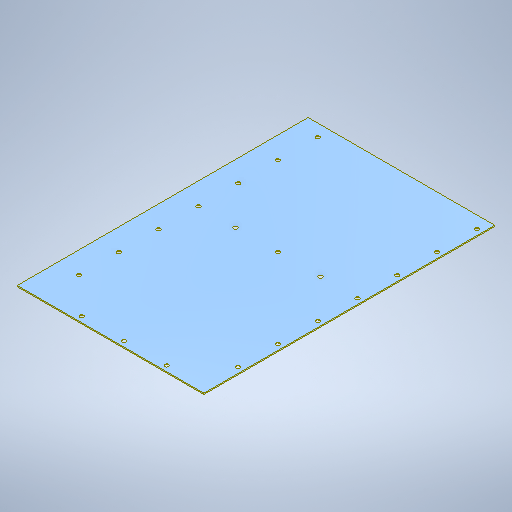
# Autodesk Inventor part: нижняя плита
Saved by Autodesk Inventor 2025 (Build 290162000, 162)
## iProperties
Created: 2025-01-21
Part Number: нижняя плита
Material: СВМПЭ, белый
Document SubType Name: Modeling
Designer: volko
Density: 0.94 g/cm^3
Appearance: Гладкий — белый
Mass: 840.848 g
Surface Area: 3697.01 cm^2
Volume: 894.519 cm^3
Author: volko
Autodesk Inventor part; units mm, degrees
ref_plane "YZ Plane" through (0, 0, 0) normal (1, 0, 0) x (0, 1, 0)
ref_plane "XZ Plane" through (0, 0, 0) normal (0, 1, 0) x (-1, 0, 0)
ref_plane "XY Plane" through (0, 0, 0) normal (0, 0, 1) x (1, 0, 0)
sketch "Эскиз1" plane through (0, 0, 0) normal (0, 1, 0) x (-1, 0, 0)
  line L0 (0, 265) -> (170, 265)
  line L1 (170, 265) -> (170, -265)
  line L2 (0, 265) -> (0, 0)
  line L3 (0, 0) -> (200, 0)
  line L4 (0, 265) -> (-170, 265)
  line L5 (-170, 265) -> (-170, -265)
  line L6 (0, -265) -> (170, -265)
  line L7 (170, -265) -> (170, -125)
  line L8 (-170, -265) -> (-170, -125)
  line L9 (0, -265) -> (-170, -265)
  point P0 (170, 125)
  point P1 (-170, 125)
  dimension "d3" = 340
  dimension "d6" = 530
  constraints: 20 end point, 7 symmetric about line, 4 point on line, 1 vertical
  measures "d3" distance between parallel lines of L5 L1
  measures "d6" distance between parallel lines of L4 L9
extrude "Выдавливание1" add sketch "Эскиз1" along normal blind 2
sketch "Эскиз2" plane through (0, 0, 0) normal (0, 1, 0) x (1, 0, 0)
  line L0 (-170, -265) -> (170, -265) projected
  line L1 (170, -265) -> (170, 265) projected
  point P0 (0, 0)
  point P1 (92.5, -255)
  point P2 (15, -255)
  point P3 (-62.5, -255)
  point P4 (92.5, 25)
  point P5 (15, 25)
  point P6 (-62.5, 25)
  point P7 (92.5, 305)
  point P8 (15, 305)
  point P9 (-62.5, 305)
  point P10 (160, -192.5)
  point P11 (160, -120)
  point P12 (160, -47.5)
  point P13 (160, 25)
  point P14 (160, 97.5)
  point P15 (160, 170)
  point P16 (160, 242.5)
  point P17 (-130, -192.5)
  point P18 (-130, -120)
  point P19 (-130, -47.5)
  point P20 (-130, 25)
  point P21 (-130, 97.5)
  point P22 (-130, 170)
  point P23 (-130, 242.5)
  dimension "d15" = 10
  dimension "d16" = 77.5
  dimension "d19" = 77.5
  dimension "d22" = 280
  dimension "d25" = 10
  dimension "d26" = 72.5
  dimension "d29" = 72.5
  dimension "d32" = 290
  constraints: 2 horizontal, 2 vertical, 21 other
  measures "d15" distance from line of L0 point (92.5, -255)
  measures "d16" distance from line of point (92.5, -255) L1
  measures "d19" distance of point (92.5, -255) point (15, -255)
  measures "d22" distance of point (92.5, -255) point (92.5, 25)
  measures "d25" distance from line of point (160, -192.5) L1
  measures "d26" distance from line of L0 point (160, -192.5)
  measures "d29" distance of point (160, -192.5) point (160, -120)
  measures "d32" distance of point (160, -192.5) point (-130, -192.5)
hole "Отверстие2" at (92.5, 0, 255) at (15, 0, 255) at (-62.5, 0, 255) at (92.5, 0, -25) at (15, 0, -25) at (-62.5, 0, -25) at (92.5, 0, -305) at (15, 0, -305) at (-62.5, 0, -305) at (160, 0, 192.5) at (160, 0, 120) at (160, 0, 47.5) at (160, 0, -25) at (160, 0, -97.5) at (160, 0, -170) at (160, 0, -242.5) at (-130, 0, 192.5) at (-130, 0, 120) at (-130, 0, 47.5) at (-130, 0, -25) at (-130, 0, -97.5) at (-130, 0, -170) at (-130, 0, -242.5) direction (0, 1, 0) diameter 3 end through all countersink diameter 11 countersink angle 90
sketch "Эскиз3" plane through (0, 0, 0) normal (0, -1, 0) x (1, 0, 0)
  line L0 (-238, 0) -> (238, 0) projected
  line L1 (0, -371) -> (0, 371) projected
  line L2 (-170, 265) -> (170, 265) projected
  point P0 (0, 0)
  point P1 (120, 207)
  point P2 (64, 207)
  point P3 (120, 235)
  point P4 (64, 235)
  point P5 (-120, 207)
  point P6 (-64, 207)
  point P7 (-120, 235)
  point P8 (-64, 235)
  point P9 (120, -207)
  point P10 (64, -207)
  point P11 (120, -235)
  point P12 (64, -235)
  point P13 (-120, -235)
  point P14 (-120, -207)
  point P15 (-64, -207)
  point P16 (-64, -235)
  dimension "d52" = 56
  dimension "d55" = 28
  dimension "d59" = 120
  dimension "d60" = 30
  constraints: 12 symmetric about line, 1 horizontal, 1 vertical, 3 other
  measures "d52" distance of point (120, 207) point (64, 207)
  measures "d55" distance of point (120, 207) point (120, 235)
  measures "d59" distance from line of L1 point (120, 207)
  measures "d60" distance from line of L2 point (120, 235)
